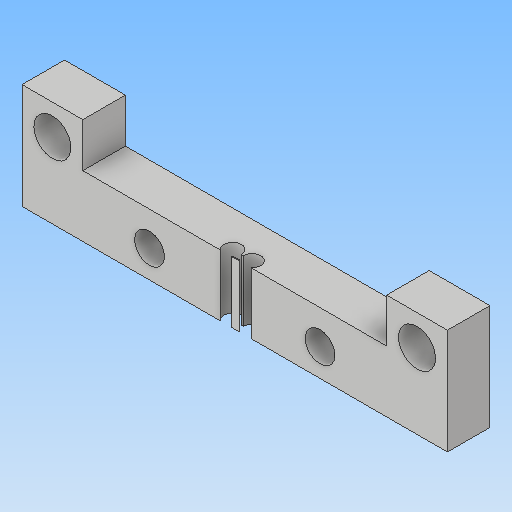
# Autodesk Inventor part: cellSTORM_inverted_sampleholder_bar
Saved by Autodesk Inventor 2019.4 (Build 234330000, 330)
## iProperties
Created: 2020-11-05
Part Number: cellSTORM_inverted_sampleholder_bar
Material: Generic
Document SubType Name: Modeling
Designer: diederichbenedict
Density: 1 g/cm^3
Appearance: Default
Author: diederichbenedict
Autodesk Inventor part; units mm, degrees
ref_plane "YZ Plane" through (0, 0, 0) normal (1, 0, 0) x (0, 1, 0)
ref_plane "XZ Plane" through (0, 0, 0) normal (0, 1, 0) x (-1, 0, 0)
ref_plane "XY Plane" through (0, 0, 0) normal (0, 0, 1) x (1, 0, 0)
sketch "Sketch1" plane through (0, 0, 0) normal (0, 0, 1) x (1, 0, 0)
  circle A0 centre (30, 26.4525) radius 3 projected
  circle A1 centre (-30, 26.4525) radius 3 projected
  line L0 (-12, 6.73) -> (12, 6.73) projected
  line L1 (12, 6.73) -> (12, 13) projected
  line L2 (12, 13) -> (-12, 13) projected
  line L3 (-12, 13) -> (-12, 6.73) projected
  line L4 (0, 33.0213) -> (0, 0)
  circle A2 centre (30, 26.4525) radius 3.05
  circle A3 centre (-30, 26.4525) radius 3.05
  line L5 (35, 31.4525) -> (35, 14.0938)
  line L6 (35, 14.0938) -> (0, 14.0938)
  line L7 (0, 24.1869) -> (25, 24.1869)
  line L8 (25, 24.1869) -> (25, 31.4525)
  line L9 (25, 31.4525) -> (35, 31.4525)
  dimension "d0" = 6.1
  dimension "d1" = 6.1
  dimension "d2" = 5
  dimension "d3" = 5
  dimension "d4" = 5
  dimension "d11" = 90
  constraints: 12 end point, 2 centre point, 2 coincident, 2 perpendicular, 2 point on line, 1 horizontal, 1 parallel, 1 vertical
  measures "d0" diameter of A2
  measures "d1" diameter of A3
  measures "d2" distance from line of A0.centre L8
  measures "d3" distance from line of A0.centre L5
  measures "d4" distance from line of A0.centre L9
  measures "d11" angle of L6 L5
extrude "Extrusion1" add sketch "Sketch1" against normal blind 7 contours L4 L7 L8 L9 L5 L6
sketch "Sketch2" plane through (0, 0, 0) normal (0, 0, 1) x (1, 0, 0)
  circle A0 centre (30, 26.4525) radius 3.05 projected
  line L0 (35, 31.4525) -> (35, 14.0938) projected
  line L1 (25, 31.4525) -> (35, 31.4525) projected
  line L2 (25, 24.1869) -> (25, 31.4525) projected
  line L3 (0, 24.1869) -> (25, 24.1869) projected
  line L4 (0, 14.0938) -> (0, 24.1869) projected
  line L5 (35, 14.0938) -> (0, 14.0938) projected
  line L6 (0, 14.0938) -> (0, 24.1869) projected
  circle A1 centre (0, 19.1403) radius 2.45
  circle A2 centre (14.0354, 18.6172) radius 2.45
  point P0 (0, 0)
  dimension "d7" = 4.9
  dimension "d8" = 4.9
  constraints: 2 centre point, 1 midpoint
  measures "d7" diameter of A1
  measures "d8" diameter of A2
extrude "Extrusion2" cut sketch "Sketch2" against normal blind 4 contours A2
mirror "Mirror1" about plane through (0, 14.0938, 0) normal (-1, 0, 0) of "Extrusion1", "Extrusion2"
sketch "Sketch3" plane through (35, 14.0938, -7) normal (0, -1, 0) x (1, 0, 0)
  line L0 (-37.45, 7) -> (-37.45, 3)
  line L1 (-40.0482, 3) -> (-44.9482, 3) projected
  line L2 (-32.55, 7) -> (-32.55, 3)
  circle A0 centre (-36.45, 5.9) radius 1.45
  circle A1 centre (-33.25, 5.9) radius 1.45
  line L3 (-35.3371, 6.8295) -> (-34.3629, 6.8295)
  line L4 (-35, 5.9) -> (-34.7, 5.9)
  point P0 (-35, 7)
  dimension "d12" = 2.9
  dimension "d13" = 2.9
  dimension "d14" = 1.1
  dimension "d15" = 0
  dimension "d16" = 3.2
  dimension "d17" = 1
  constraints: 8 end point, 4 point on circle, 2 centre point, 2 vertical, 1 horizontal, 1 parallel, 3 other
  measures "d12" diameter of A0
  measures "d13" diameter of A1
  measures "d14" vertical distance of A0.centre L0.start
  measures "d15" vertical distance of A0.centre A1.centre
  measures "d16" distance of A1.centre A0.centre
  measures "d17" distance from line of A0.centre L0
extrude "Extrusion3" cut sketch "Sketch3" against normal through all
body "Solid1"
